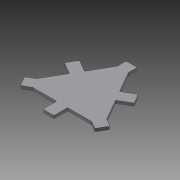
# Autodesk Inventor part: Frame_Bed
Saved by Autodesk Inventor 2014 (Build 180170000, 170)
## iProperties
Created: 2014-08-27
Part Number: Frame_Bed
Material: Generic
Document SubType Name: Modeling
Designer: ThatOtherGuy
Density: 1 g/cm^3
Appearance: Default
Author: ThatOtherGuy
Autodesk Inventor part; units mm, degrees
ref_plane "YZ Plane" through (0, 0, 0) normal (1, 0, 0) x (0, 1, 0)
ref_plane "XZ Plane" through (0, 0, 0) normal (0, 1, 0) x (-1, 0, 0)
ref_plane "XY Plane" through (0, 0, 0) normal (0, 0, 1) x (1, 0, 0)
sketch "Sketch2" plane through (0, 0, 0) normal (0, 0, 1) x (1, 0, 0)
  line L0 (0, 0) -> (-63.75, 36.8061)
  line L1 (63.75, 36.8061) -> (0, 0)
  line L2 (0, 0) -> (147.7389, 0) construction
  line L3 (63.75, 36.8061) -> (42.5, 73.6122)
  line L4 (-42.5, 73.6122) -> (-63.75, 36.8061)
  line L5 (-42.5, 73.6122) -> (42.5, 73.6122)
  line L6 (-12.5, 73.6122) -> (-12.5, 105)
  line L7 (12.5, 105) -> (12.5, 73.6122)
  line L8 (63.75, 36.8061) -> (85, 0) construction
  line L9 (12.5, 88.6122) -> (27.5, 73.6122)
  line L10 (-27.5, 73.6122) -> (-12.5, 88.6122)
  line L11 (63.75, 36.8061) -> (77.9423, 45)
  line L12 (77.9423, 45) -> (61.423, 73.6122)
  line L13 (61.423, 73.6122) -> (42.5, 73.6122)
  line L14 (-63.75, 36.8061) -> (-77.9423, 45)
  line L15 (-77.9423, 45) -> (-61.423, 73.6122)
  line L16 (-61.423, 73.6122) -> (-42.5, 73.6122)
  line L17 (-12.5, 105) -> (12.5, 105)
  dimension "d29" = 120
  dimension "d30" = 30
  dimension "d31" = 30
  dimension "d33" = 25
  dimension "d34" = 85
  dimension "d35" = 60
  dimension "d36" = 85
  dimension "d37" = 45
  dimension "d38" = 15
  dimension "d45" = 90
  dimension "d47" = 105
  constraints: 36 end point, 8 perpendicular, 7 point on line, 5 equal length, 2 collinear, 2 parallel, 1 horizontal
  measures "d29" angle of L0 L1
  measures "d30" angle of L2 L1
  measures "d31" angle of L2 L0
  measures "d33" distance between parallel lines of L6 L7
  measures "d34" distance of L4.start L3.end
  measures "d35" angle of L2 L3
  measures "d36" distance of L8.end L3.end
  measures "d37" angle of L5 L9
  measures "d38" distance of L7.end L9.start
  measures "d45" distance of L11.end L0.start
  measures "d47" distance from line of L0.start L17
extrude "Extrusion2" add sketch "Sketch2" along normal blind 6.731
fillet "Fillet3" radius 1.5875 8 edges at (61.423, 73.6122, 3.3655) (27.5, 73.6122, 3.3655) (12.5, 88.6122, 3.3655) (12.5, 105, 3.3655) (-12.5, 88.6122, 3.3655) (-27.5, 73.6122, 3.3655) (-61.423, 73.6122, 3.3655) (-12.5, 105, 3.3655)
pattern_circular "Circular Pattern1" count 3 over 360 about axis through (0, 0, 0) along (0, 0, 1) of "Extrusion2", "Fillet3"
equation "\"d30\" = d31"
equation "\"d36\" = d34"
equation "\"d39\" = THICKB"
equation "\"THICKA\" = 3.175"
equation "\"THICKB\" = 6.731"
equation "\"THICKC\" = 12.7"
equation "\"BALLDIA\" = 12"
equation "\"MAGDIA\" = 9.5"
equation "\"THICKPLY\" = 5"
body "Solid2"
